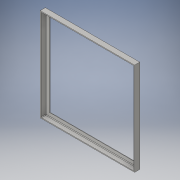
# Autodesk Inventor part: rackTop
Saved by Autodesk Inventor 2016 (Build 200138000, 138)
## iProperties
Created: 2016-08-03
Part Number: rackTop
Material: Generic
Document SubType Name: Modeling
Designer: Zuhra Abdurashidova
Density: 1 g/cm^3
Appearance: Default
Author: Zuhra Abdurashidova
Autodesk Inventor part; units mm, degrees
ref_plane "YZ Plane" through (0, 0, 0) normal (1, 0, 0) x (0, 1, 0)
ref_plane "XZ Plane" through (0, 0, 0) normal (0, 1, 0) x (-1, 0, 0)
ref_plane "XY Plane" through (0, 0, 0) normal (0, 0, 1) x (1, 0, 0)
sketch "Sketch1" plane through (0, 0, 0) normal (0, 0, 1) x (1, 0, 0)
  line L0 (-257.9687, -254) -> (257.9688, -254)
  line L1 (257.9688, -254) -> (257.9687, 254)
  line L2 (257.9687, 254) -> (-257.9688, 254)
  line L3 (-257.9688, 254) -> (-257.9687, -254)
  line L4 (-257.9687, -254) -> (257.9687, 254) construction
  line L5 (257.9688, -254) -> (-257.9688, 254) construction
  line L6 (232.5688, -228.6) -> (-232.5687, -228.6)
  line L7 (-232.5687, -228.6) -> (-232.5688, 228.6)
  line L8 (-232.5688, 228.6) -> (232.5687, 228.6)
  line L9 (232.5687, 228.6) -> (232.5688, -228.6)
  point P0 (0, 0)
  dimension "d0" = 515.9375
  dimension "d1" = 508
  dimension "d2" = 25.4
  constraints: 20 end point, 4 parallel, 2 midpoint, 2 perpendicular, 1 horizontal, 3 other
  measures "d0" distance of L0.start L0.end
  measures "d1" distance of L0.end L1.end
  measures "d2" distance between parallel lines of L6 L0
extrude "Extrusion1" add sketch "Sketch1" along normal blind 2.6568
sketch "Sketch2" plane through (0, 0, 2.6568) normal (0, 0, 1) x (1, 0, 0)
  line L0 (-257.9688, 254) -> (-257.9687, -254) projected
  line L1 (-257.9688, 254) -> (257.9688, 254)
  line L2 (257.9688, 254) -> (257.9688, -254)
  line L3 (257.9688, -254) -> (-257.9688, -254)
  line L4 (-257.9688, -254) -> (-257.9688, 254)
  line L5 (-253.3831, -249.4144) -> (253.3831, -249.4144)
  line L6 (253.3831, -249.4144) -> (253.3831, 249.4144)
  line L7 (253.3831, 249.4144) -> (-253.3831, 249.4144)
  line L8 (-253.3831, 249.4144) -> (-253.3831, -249.4144)
  point P0 (0, 0)
  constraints: 16 end point, 4 parallel, 2 perpendicular, 1 horizontal, 3 other
extrude "Extrusion2" add sketch "Sketch2" along normal blind 25.4
fillet "Fillet1" radius 3.175 8 edges at (-253.3831, 0, 2.6568) (0, -249.4144, 2.6568) (-253.3831, -249.4144, 15.3568) (253.3831, 0, 2.6568) (253.3831, -249.4144, 15.3568) (0, 249.4144, 2.6568) (253.3831, 249.4144, 15.3568) (-253.3831, 249.4144, 15.3568)
body "Solid1"
